Autodesk Inventor part; units mm, degrees
(part 2 of 2)
  arc A228 (-0.5092, 0) -> (-0.3793, 0.075) centre (-0.5092, 0.15) ccw
  arc A229 (-0.1195, 0.075) -> (0.0104, 0) centre (0.0104, 0.15) ccw
  arc A230 (-0.1195, 0.075) -> (-0.3793, 0.075) centre (-0.2494, 0) ccw
  point P0 (10, 28.3)
  point P1 (-0.5092, 0)
  point P2 (-1.0289, 0)
  point P3 (-1.5485, 0)
  point P4 (-2.0681, 0)
  point P5 (-2.5877, 0)
  point P6 (-3.1073, 0)
  point P7 (-3.6269, 0)
  point P8 (-4.1465, 0)
  point P9 (-4.6662, 0)
  point P10 (-5.1858, 0)
  point P11 (-5.7054, 0)
  point P12 (-6.225, 0)
  point P13 (-6.7446, 0)
  point P14 (-7.2642, 0)
  point P15 (-7.7839, 0)
  point P16 (-8.3035, 0)
  point P17 (-8.8231, 0)
  point P18 (-9.3427, 0)
  point P19 (-9.8623, 0)
  point P20 (-10.3819, 0)
  point P21 (-10.9015, 0)
  point P22 (-11.4212, 0)
  point P23 (-11.9408, 0)
  point P24 (-12.4604, 0)
  point P25 (-12.98, 0)
  point P26 (-13.4996, 0)
  point P27 (-14.0192, 0)
  point P28 (-14.5389, 0)
  point P29 (-15.0585, 0)
  point P30 (-15.5781, 0)
  point P31 (-16.0977, 0)
  point P32 (-16.6173, 0)
  point P33 (-17.1369, 0)
  point P34 (-17.6565, 0)
  point P35 (-18.1762, 0)
  point P36 (-18.6958, 0)
  point P37 (-19.2154, 0)
  point P38 (-19.735, 0)
  point P39 (-20.2546, 0)
  point P40 (-20.7742, 0)
  point P41 (-21.2939, 0)
  point P42 (-21.8135, 0)
  point P43 (-22.3331, 0)
  point P44 (-22.8527, 0)
  point P45 (-23.3723, 0)
  point P46 (-23.8919, 0)
  point P47 (-24.4115, 0)
  point P48 (-24.9312, 0)
  point P49 (-25.4508, 0)
  point P50 (-25.9704, 0)
  point P51 (-26.49, 0)
  point P52 (-27.0096, 0)
  point P53 (-27.5292, 0)
  point P54 (-28.0488, 0)
  point P55 (-28.5685, 0)
  point P56 (-29.0881, 0)
  point P57 (-29.6077, 0)
  point P58 (-30.1273, 0)
  point P59 (-30.6469, 0)
  point P60 (-31.1665, 0)
  point P61 (-31.6862, 0)
  point P62 (-32.2058, 0)
  point P63 (-32.7254, 0)
  point P64 (-33.245, 0)
  point P65 (-33.7646, 0)
  point P66 (-34.2842, 0)
  point P67 (-34.8038, 0)
  point P68 (-35.3235, 0)
  point P69 (-35.8431, 0)
  point P70 (-36.3627, 0)
  point P71 (-36.8823, 0)
  point P72 (-37.4019, 0)
  point P73 (-37.9215, 0)
  point P74 (-38.4412, 0)
  point P75 (-38.9608, 0)
  point P76 (-39.4804, 0)
  dimension "d85" = 0.5196
  dimension "d88" = 0.5196
  constraints: 462 point on circle, 231 centre point, 1 horizontal, 836 other
  measures "d85" distance of A0.start A2.end
  measures "d88" distance of A0.centre A3.centre
sketch3d "3D Sketch1"
sweep "Sweep1" [suppressed]
chamfer "Chamfer5" distance 0.5 angle 45 32 edges at (-28.2, 60, 0) (-26.838, 60, 26.838) (-28.2, 60, 21.325) (-28.2, 60, -21.325) (0, 60, 28.2) (26.838, 60, 26.838) (28.2, 60, 21.325) (28.2, 60, 0) (28.2, 60, -21.325) (26.838, 60, -26.838) (0, 60, -28.2) (-26.838, 60, -26.838) (0, 0, 28.2) (18.1213, 0, 27.3213) (19, 0, 23.6) (23.6, 0, 19) (27.3213, 0, 18.1213) (28.2, 0, 0) (27.3213, 0, -18.1213) (23.6, 0, -19) (19, 0, -23.6) (18.1213, 0, -27.3213) (0, 0, -28.2) (-18.1213, 0, -27.3213) (-19, 0, -23.6) (-23.6, 0, -19) (-27.3213, 0, -18.1213) (-28.2, 0, 0) (-27.3213, 0, 18.1213) (-23.6, 0, 19) (-19, 0, 23.6) (-18.1213, 0, 27.3213)
equation "\"d9\" = d10"
equation "\"d10\" = 0.5 * d7"
equation "\"d21\" = d20"
equation "\"d67\" = d66"
equation "\"d69\" = 0.5 * d67"
equation "\"d70\" = 0.5 * d67"
equation "\"d80\" = d77"
body "Solid1"
